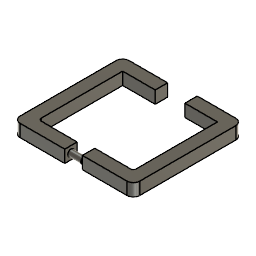
bot_mounts_1 (Autodesk Fusion 360 design; units mm, degrees)
part number: 2025-11-27-19-44-46-816
part number: 2025-11-27-20-02-49-671
part number: 2025-11-27-20-02-49-676
Autodesk Fusion 360 part; units mm, degrees
sketch "Sketch1" plane through (0, 0, 0) normal (1, 0, 0) x (0, 1, 0)
  line L0 (0, 0) -> (9.7, 0)
  line L1 (9.7, 0) -> (9.7, 9.7)
  line L2 (9.7, 9.7) -> (0, 9.7)
  line L3 (0, 9.7) -> (0, 0)
  dimension "d1" = 9.7
  dimension "d2" = 9.7
  constraint horizontal L0
  constraint vertical L1
  constraint horizontal L2
  constraint vertical L3
  constraint coincident L0.start L3.end
  measures "d1" distance of L0.start L0.end
  measures "d2" distance of L0.start L2.end
extrude "Extrude1" add sketch "Sketch1" along normal blind 40 makes body 1
sketch "Sketch2" plane through (0, 0, 0) normal (0, -1, 0) x (1, 0, 0)
  line L0 (0, 9.7) -> (0, 0)
  line L1 (0, 0) -> (40, 0)
  line L2 (40, 0) -> (40, 9.7)
  line L3 (40, 9.7) -> (0, 9.7)
  line L4 (40, 9.7) -> (30.3, 9.7)
  line L5 (30.3, 9.7) -> (30.3, 0)
  line L6 (30.3, 0) -> (40, 0)
  line L7 (40, 0) -> (40, 9.7)
  dimension "d5" = 9.7
  constraint horizontal L4
  constraint vertical L5
  constraint horizontal L6
  constraint vertical L7
  constraint coincident L2.end L3.start
  measures "d5" distance of L2.end L4.end
extrude "Extrude2" add sketch "Sketch2" along normal blind 75 contours L1 L2 L3 L4 L5 L6 L7 bodies 1
sketch "Sketch3" plane through (30.3, 0, 0) normal (-1, 0, 0) x (0, -1, 0)
  line L0 (0, 9.7) -> (0, 0)
  line L1 (0, 0) -> (75, 0)
  line L2 (75, 0) -> (75, 9.7)
  line L3 (75, 9.7) -> (0, 9.7)
  line L4 (75, 9.7) -> (65.3, 9.7)
  line L5 (65.3, 9.7) -> (65.3, -2.721)
  line L6 (65.3, -2.721) -> (75, -2.721)
  line L7 (75, -2.721) -> (75, 9.7)
  dimension "d8" = 9.7
  constraint horizontal L4
  constraint vertical L5
  constraint horizontal L6
  constraint vertical L7
  constraint coincident L2.end L3.start
  measures "d8" distance of L2.end L4.end
extrude "Extrude3" add sketch "Sketch3" along normal blind 30 contours L1 L2 L3 L4 L5 L7 bodies 1
sketch "Sketch4" plane through (0.3, 0, 0) normal (-1, 0, 0) x (0, -1, 0)
  line L0 (75, 0) -> (75, 9.7)
  line L1 (75, 9.7) -> (65.3, 9.7)
  line L2 (65.3, 9.7) -> (65.3, 0)
  line L3 (65.3, 0) -> (75, 0)
  circle A0 centre (70.15, 4.85) radius 2.5
  line L4 (70.15, 9.7) -> (70.15, 0)
  line L5 (65.3, 4.85) -> (75, 4.85)
  dimension "d11" = 5
  constraint midpoint L1 L4.start
  constraint midpoint L3 L4.end
  constraint midpoint L2 L5.start
  constraint midpoint L0 L5.end
  constraint midpoint A0.centre L4
  measures "d11" diameter of A0
extrude "Extrude5" cut sketch "Sketch4" along normal mid plane 20 contours A0 L4 L5 | A0 L4 L5 | A0 L4 L5 | A0 L4 L5 bodies 1
mirror "Mirror1" about plane through (0, 0, 0) normal (1, 0, 0) of bodies 1 makes body 2
extrude "Extrude6" add sketch "Sketch4" along normal up to surface (10.6 mm away) and the other way blind 10 contours A0 L4 L5 | A0 L4 L5 | A0 L4 L5 | A0 L4 L5 bodies 2
chamfer "Chamfer1" distance 0.5 angle 45 1 edges at (10.3, -67.8192, 5.754) on bodies 2
copy_body "Body->Comp1" bodies 1 removing the originals makes body 3 in component "Component"
copy_body "Body->Comp2" bodies 2 removing the originals makes body 4 in component "Component'"
move_face "OffsetFaces1" offset -0.15 1 faces at (3.6333, -72.6376, 5.0989) on bodies 3 in component "Component"
extrude "Extrude1'" cut 1 faces at (0, 3.2333, 6.4667) along direction (1, 0, 0) blind 5 on bodies 3 bodies 3 in component "Component"
extrude "Extrude1''" cut 1 faces at (0, 3.2333, 6.4667) along direction (-1, 0, 0) blind 5 on bodies 4 bodies 4 in component "Component'"
fillet "Fillet1" radius 2 1 edges at (30.3, -65.3, 4.85) on bodies 3 in component "Component"
fillet "Fillet1'" radius 2 1 edges at (-30.3, -65.3, 4.85) on bodies 4 in component "Component'"
fillet "Fillet2" radius 5 1 edges at (40, -75, 4.85) on bodies 3 in component "Component"
fillet "Fillet2'" radius 5 1 edges at (-40, -75, 4.85) on bodies 4 in component "Component'"
fillet "Fillet3" radius 5 1 edges at (40, 9.7, 4.85) on bodies 3 in component "Component"
fillet "Fillet3'" radius 5 1 edges at (-40, 9.7, 4.85) on bodies 4 in component "Component'"
component "Component" placed x (1, 0, 0) y (0, 1, 0) z (0, 0, 1) at (0, 0, 0)
component "Component'" placed x (1, 0, 0) y (0, 1, 0) z (0, 0, 1) at (-17.0193, 3.9794, -6.6227)
